Autodesk Fusion 360 part; units mm, degrees
(part 2 of 3)
  line L394 (91.6491, -63.7888) -> (96.0664, -64.6474)
  spline S217 degree 3 poles (106.4792, -50.6897) (105.7323, -50.6279) (105.0622, -51.1477) (104.9365, -51.8866) knots 0 0 0 0 1 1 1 1
  spline S218 degree 3 poles (7.9042, -66.3389) (7.576, -66.0107) (7.3916, -65.5656) (7.3916, -65.1015) knots 0 0 0 0 1 1 1 1
  spline S219 degree 3 poles (32.1681, -40.899) (31.7818, -41.2853) (31.2578, -41.5024) (30.7115, -41.5024) knots 0 0 0 0 1 1 1 1
  line L395 (26.4924, -39.9217) -> (26.4924, -39.9217)
  line L396 (96.8435, -63.2704) -> (97.4297, -62.875)
  line L397 (111.9353, -56.4836) -> (110.6261, -56.4379)
  spline S220 degree 3 poles (28.6515, -39.4424) (28.6515, -38.896) (28.8685, -38.372) (29.2548, -37.9857) knots 0 0 0 0 1 1 1 1
  line L398 (100.2141, -70.0378) -> (98.6435, -69.7326)
  spline S221 degree 3 poles (26.1234, -39.0308) (26.3597, -39.2671) (26.4924, -39.5875) (26.4924, -39.9217) knots 0 0 0 0 1 1 1 1
  spline S222 degree 3 poles (29.2548, -40.899) (28.8685, -40.5127) (28.6515, -39.9887) (28.6515, -39.4424) knots 0 0 0 0 1 1 1 1
  spline S223 degree 3 poles (36.1906, -40.223) (35.8564, -40.223) (35.5359, -40.0903) (35.2996, -39.854) knots 0 0 0 0 1 1 1 1
  line L399 (97.4297, -62.875) -> (102.3378, -63.829)
  line L400 (96.6527, -64.252) -> (96.8435, -63.2704)
  line L401 (103.1261, -76.3087) -> (101.8401, -76.0587)
  spline S224 degree 3 poles (103.4983, -45.9378) (103.5956, -45.8471) (103.6523, -45.721) (103.6556, -45.588) knots 0 0 0 0 1 1 1 1
  line L402 (31.7998, -44.3662) -> (30.4948, -44.4804)
  spline S225 degree 3 poles (37.0815, -38.072) (37.3178, -38.3083) (37.4506, -38.6288) (37.4506, -38.963) knots 0 0 0 0 1 1 1 1
  spline S226 degree 3 poles (7.3916, -65.1015) (7.3916, -64.6373) (7.576, -64.1922) (7.9042, -63.864) knots 0 0 0 0 1 1 1 1
  spline S227 degree 3 poles (112.8027, -57.4145) (112.8201, -56.918) (112.4318, -56.5013) (111.9353, -56.4836) knots 0 0 0 0 1 1 1 1
  spline S228 degree 3 poles (10.3791, -63.864) (10.7073, -64.1922) (10.8916, -64.6373) (10.8916, -65.1015) knots 0 0 0 0 1 1 1 1
  line L403 (102.749, -64.4387) -> (102.6575, -64.9098)
  spline S229 degree 3 poles (111.584, -35.6994) (111.8203, -35.4631) (112.1408, -35.3303) (112.4749, -35.3303) knots 0 0 0 0 1 1 1 1
  line L404 (38.9322, -55.8983) -> (38.9322, -55.8983)
  spline S230 degree 3 poles (29.2548, -37.9857) (29.6412, -37.5994) (30.1651, -37.3824) (30.7115, -37.3824) knots 0 0 0 0 1 1 1 1
  line L405 (32.7715, -39.4424) -> (32.7715, -39.4424)
  spline S231 degree 3 poles (37.6722, -57.1583) (37.338, -57.1583) (37.0175, -57.0256) (36.7812, -56.7893) knots 0 0 0 0 1 1 1 1
  spline S232 degree 3 poles (107.3956, -43.2171) (107.8921, -43.2341) (108.3085, -42.8455) (108.3258, -42.349) knots 0 0 0 0 1 1 1 1
  spline S233 degree 3 poles (85.5554, -23.6785) (85.6511, -23.5861) (85.7056, -23.4591) (85.7065, -23.3261) knots 0 0 0 0 1 1 1 1
  spline S234 degree 3 poles (111.2149, -36.5903) (111.2149, -36.2562) (111.3477, -35.9357) (111.584, -35.6994) knots 0 0 0 0 1 1 1 1
  spline S235 degree 3 poles (32.1681, -37.9857) (32.5545, -38.372) (32.7715, -38.896) (32.7715, -39.4424) knots 0 0 0 0 1 1 1 1
  spline S236 degree 3 poles (36.7812, -55.0074) (37.0175, -54.7711) (37.338, -54.6383) (37.6722, -54.6383) knots 0 0 0 0 1 1 1 1
  spline S237 degree 3 poles (85.1979, -23.8173) (85.3309, -23.8209) (85.4597, -23.7709) (85.5554, -23.6785) knots 0 0 0 0 1 1 1 1
  spline S238 degree 3 poles (33.6498, -54.921) (34.0361, -55.3074) (34.2531, -55.8313) (34.2531, -56.3777) knots 0 0 0 0 1 1 1 1
  spline S239 degree 3 poles (30.7115, -41.5024) (30.1651, -41.5024) (29.6412, -41.2853) (29.2548, -40.899) knots 0 0 0 0 1 1 1 1
  line L406 (85.724, -22.3262) -> (86.2326, -21.835)
  line L407 (107.4584, -41.4182) -> (106.1492, -41.3725)
  line L408 (87.0806, -30.5511) -> (87.0972, -29.6013)
  spline S240 degree 3 poles (113.7349, -36.5903) (113.7349, -36.9245) (113.6022, -37.245) (113.3659, -37.4813) knots 0 0 0 0 1 1 1 1
  line L409 (94.2137, -27.5752) -> (91.1841, -27.5223)
  line L410 (85.7065, -23.3261) -> (85.724, -22.3262)
  spline S241 degree 3 poles (30.7365, -54.921) (31.1228, -54.5347) (31.6468, -54.3177) (32.1931, -54.3177) knots 0 0 0 0 1 1 1 1
  spline S242 degree 3 poles (105.219, -42.2406) (105.2016, -42.7371) (105.5899, -43.1537) (106.0864, -43.1714) knots 0 0 0 0 1 1 1 1
  line L411 (34.2531, -56.3777) -> (34.2531, -56.3777)
  spline S243 degree 3 poles (38.5632, -56.7893) (38.3269, -57.0256) (38.0064, -57.1583) (37.6722, -57.1583) knots 0 0 0 0 1 1 1 1
  line L412 (86.2326, -21.835) -> (91.2319, -21.9223)
  spline S244 degree 3 poles (38.9322, -55.8983) (38.9322, -56.2325) (38.7995, -56.553) (38.5632, -56.7893) knots 0 0 0 0 1 1 1 1
  line L413 (90.2186, -28.4056) -> (88.6188, -28.3777)
  spline S245 degree 3 poles (30.7115, -37.3824) (31.2578, -37.3824) (31.7818, -37.5994) (32.1681, -37.9857) knots 0 0 0 0 1 1 1 1
  line L414 (91.1841, -27.5223) -> (90.2186, -28.4056)
  line L415 (87.0806, -30.5511) -> (80.5816, -30.4377)
  spline S246 degree 3 poles (106.1492, -41.3725) (105.6527, -41.3555) (105.2363, -41.744) (105.219, -42.2406) knots 0 0 0 0 1 1 1 1
  line L416 (80.5982, -29.4878) -> (78.0236, -29.4429)
  line L417 (78.0236, -29.4429) -> (78.1039, -24.8436)
  spline S247 degree 3 poles (37.6722, -54.6383) (38.0064, -54.6383) (38.3269, -54.7711) (38.5632, -55.0074) knots 0 0 0 0 1 1 1 1
  spline S248 degree 3 poles (113.3659, -37.4813) (113.1296, -37.7176) (112.8091, -37.8503) (112.4749, -37.8503) knots 0 0 0 0 1 1 1 1
  line L418 (80.6986, -23.7387) -> (85.1979, -23.8173)
  spline S249 degree 3 poles (89.4046, -20.8902) (89.9013, -20.8984) (90.3106, -20.5027) (90.3193, -20.0061) knots 0 0 0 0 1 1 1 1
  spline S250 degree 3 poles (88.6188, -28.3777) (87.8709, -28.3289) (87.21, -28.8604) (87.0972, -29.6013) knots 0 0 0 0 1 1 1 1
  line L419 (89.4046, -20.8902) -> (88.0948, -20.8674)
  spline S251 degree 3 poles (90.3193, -20.0061) (90.328, -19.5094) (89.9326, -19.0997) (89.436, -19.0905) knots 0 0 0 0 1 1 1 1
  spline S252 degree 3 poles (87.2115, -19.9518) (87.2029, -20.4485) (87.5982, -20.8582) (88.0948, -20.8674) knots 0 0 0 0 1 1 1 1
  spline S253 degree 3 poles (111.584, -37.4813) (111.3477, -37.245) (111.2149, -36.9245) (111.2149, -36.5903) knots 0 0 0 0 1 1 1 1
  spline S254 degree 3 poles (88.1262, -19.0676) (87.6296, -19.0595) (87.2202, -19.4552) (87.2115, -19.9518) knots 0 0 0 0 1 1 1 1
  spline S255 degree 3 poles (112.4749, -37.8503) (112.1408, -37.8503) (111.8203, -37.7176) (111.584, -37.4813) knots 0 0 0 0 1 1 1 1
  spline S256 degree 3 poles (36.4122, -55.8983) (36.4122, -55.5641) (36.545, -55.2437) (36.7812, -55.0074) knots 0 0 0 0 1 1 1 1
  line L420 (80.5816, -30.4377) -> (80.5982, -29.4878)
  spline S257 degree 3 poles (38.5632, -55.0074) (38.7995, -55.2437) (38.9322, -55.5641) (38.9322, -55.8983) knots 0 0 0 0 1 1 1 1
  line L421 (107.3956, -43.2171) -> (106.0864, -43.1714)
  line L422 (80.6785, -24.8885) -> (80.6986, -23.7387)
  line L423 (78.1039, -24.8436) -> (80.6785, -24.8885)
  line L424 (91.7343, -22.9312) -> (94.294, -22.9759)
  spline S258 degree 3 poles (108.3258, -42.349) (108.3431, -41.8525) (107.9549, -41.4359) (107.4584, -41.4182) knots 0 0 0 0 1 1 1 1
  spline S259 degree 3 poles (90.9284, -14.0798) (90.9284, -14.6262) (90.7113, -15.1501) (90.325, -15.5365) knots 0 0 0 0 1 1 1 1
  spline S260 degree 3 poles (90.325, -15.5365) (89.9387, -15.9228) (89.4147, -16.1398) (88.8684, -16.1398) knots 0 0 0 0 1 1 1 1
  line L425 (91.7427, -22.4513) -> (91.7343, -22.9312)
  spline S261 degree 3 poles (36.7812, -56.7893) (36.545, -56.553) (36.4122, -56.2325) (36.4122, -55.8983) knots 0 0 0 0 1 1 1 1
  line L426 (94.2137, -27.5752) -> (94.294, -22.9759)
  spline S262 degree 3 poles (88.8684, -16.1398) (88.322, -16.1398) (87.7981, -15.9228) (87.4117, -15.5365) knots 0 0 0 0 1 1 1 1
  spline S263 degree 3 poles (87.4117, -15.5365) (87.0254, -15.1501) (86.8084, -14.6262) (86.8084, -14.0798) knots 0 0 0 0 1 1 1 1
  spline S264 degree 3 poles (88.8684, -12.0198) (89.4147, -12.0198) (89.9387, -12.2369) (90.325, -12.6232) knots 0 0 0 0 1 1 1 1
  spline S265 degree 3 poles (86.8084, -14.0798) (86.8084, -12.9421) (87.7307, -12.0198) (88.8684, -12.0198) knots 0 0 0 0 1 1 1 1
  spline S266 degree 3 poles (32.1931, -54.3177) (32.7395, -54.3177) (33.2634, -54.5347) (33.6498, -54.921) knots 0 0 0 0 1 1 1 1
  line L427 (89.436, -19.0905) -> (88.1262, -19.0676)
  line L428 (91.2319, -21.9223) -> (91.7427, -22.4513)
  spline S267 degree 3 poles (82.1092, -13.9838) (82.1092, -13.6497) (82.242, -13.3292) (82.4783, -13.0929) knots 0 0 0 0 1 1 1 1
  spline S268 degree 3 poles (94.0709, -32.4332) (93.7367, -32.4332) (93.4162, -32.3005) (93.1799, -32.0642) knots 0 0 0 0 1 1 1 1
  line L429 (95.3309, -31.1732) -> (95.3309, -31.1732)
  spline S269 degree 3 poles (94.9618, -30.2823) (95.1981, -30.5186) (95.3309, -30.8391) (95.3309, -31.1732) knots 0 0 0 0 1 1 1 1
  spline S270 degree 3 poles (11.2142, -14.5989) (10.886, -14.2707) (10.7016, -13.8256) (10.7016, -13.3615) knots 0 0 0 0 1 1 1 1
  spline S271 degree 3 poles (11.2142, -12.124) (11.5424, -11.7958) (11.9875, -11.6115) (12.4516, -11.6115) knots 0 0 0 0 1 1 1 1
  spline S272 degree 3 poles (10.3791, -66.3389) (10.0509, -66.6671) (9.6058, -66.8515) (9.1416, -66.8515) knots 0 0 0 0 1 1 1 1
  spline S273 degree 3 poles (84.6292, -13.9838) (84.6292, -14.318) (84.4965, -14.6385) (84.2602, -14.8748) knots 0 0 0 0 1 1 1 1
  spline S274 degree 3 poles (90.6317, -31.0772) (90.6317, -31.6236) (90.4147, -32.1476) (90.0283, -32.5339) knots 0 0 0 0 1 1 1 1
  spline S275 degree 3 poles (93.4766, -13.2849) (93.7129, -13.0486) (94.0334, -12.9158) (94.3675, -12.9158) knots 0 0 0 0 1 1 1 1
  spline S276 degree 3 poles (88.5717, -29.0172) (89.118, -29.0172) (89.642, -29.2343) (90.0283, -29.6206) knots 0 0 0 0 1 1 1 1
  line L430 (89.1393, -36.0879) -> (87.8295, -36.0651)
  spline S277 degree 3 poles (88.5717, -33.1372) (88.0254, -33.1372) (87.5014, -32.9202) (87.1151, -32.5339) knots 0 0 0 0 1 1 1 1
  spline S278 degree 3 poles (81.8125, -30.9813) (81.8125, -30.6471) (81.9453, -30.3266) (82.1816, -30.0903) knots 0 0 0 0 1 1 1 1
  spline S279 degree 3 poles (87.1151, -29.6206) (87.5014, -29.2343) (88.0254, -29.0172) (88.5717, -29.0172) knots 0 0 0 0 1 1 1 1
  line L431 (90.9284, -14.0798) -> (90.9284, -14.0798)
  line L432 (90.6317, -31.0772) -> (90.6317, -31.0772)
  spline S280 degree 3 poles (95.2585, -13.2849) (95.4948, -13.5212) (95.6275, -13.8416) (95.6275, -14.1758) knots 0 0 0 0 1 1 1 1
  line L433 (84.6292, -13.9838) -> (84.6292, -13.9838)
  spline S281 degree 3 poles (94.0709, -29.9132) (94.405, -29.9132) (94.7255, -30.046) (94.9618, -30.2823) knots 0 0 0 0 1 1 1 1
  spline S282 degree 3 poles (10.7016, -13.3615) (10.7016, -12.8973) (10.886, -12.4522) (11.2142, -12.124) knots 0 0 0 0 1 1 1 1
  spline S283 degree 3 poles (14.8422, -46.7533) (14.7989, -46.2586) (14.363, -45.8924) (13.8683, -45.935) knots 0 0 0 0 1 1 1 1
  spline S284 degree 3 poles (83.3692, -15.2438) (83.0351, -15.2438) (82.7146, -15.1111) (82.4783, -14.8748) knots 0 0 0 0 1 1 1 1
  spline S285 degree 3 poles (94.3675, -15.4358) (94.0334, -15.4358) (93.7129, -15.3031) (93.4766, -15.0668) knots 0 0 0 0 1 1 1 1
  spline S286 degree 3 poles (9.1416, -66.8515) (8.6775, -66.8515) (8.2324, -66.6671) (7.9042, -66.3389) knots 0 0 0 0 1 1 1 1
  spline S287 degree 3 poles (10.8916, -65.1015) (10.8916, -65.5656) (10.7073, -66.0107) (10.3791, -66.3389) knots 0 0 0 0 1 1 1 1
  spline S288 degree 3 poles (89.1079, -37.8876) (89.6046, -37.8958) (90.0139, -37.5001) (90.0226, -37.0035) knots 0 0 0 0 1 1 1 1
  spline S289 degree 3 poles (86.9148, -36.9492) (86.9062, -37.4459) (87.3015, -37.8556) (87.7981, -37.8648) knots 0 0 0 0 1 1 1 1
  spline S290 degree 3 poles (82.1816, -30.0903) (82.4179, -29.854) (82.7384, -29.7213) (83.0725, -29.7213) knots 0 0 0 0 1 1 1 1
  spline S291 degree 3 poles (94.9618, -32.0642) (94.7255, -32.3005) (94.405, -32.4332) (94.0709, -32.4332) knots 0 0 0 0 1 1 1 1
  spline S292 degree 3 poles (95.2585, -15.0668) (95.0222, -15.3031) (94.7017, -15.4358) (94.3675, -15.4358) knots 0 0 0 0 1 1 1 1
  spline S293 degree 3 poles (90.325, -12.6232) (90.7113, -13.0095) (90.9284, -13.5335) (90.9284, -14.0798) knots 0 0 0 0 1 1 1 1
  spline S294 degree 3 poles (82.1816, -31.8722) (81.9453, -31.6359) (81.8125, -31.3154) (81.8125, -30.9813) knots 0 0 0 0 1 1 1 1
  spline S295 degree 3 poles (93.1799, -30.2823) (93.4162, -30.046) (93.7367, -29.9132) (94.0709, -29.9132) knots 0 0 0 0 1 1 1 1
  spline S296 degree 3 poles (83.9635, -31.8722) (83.7272, -32.1085) (83.4067, -32.2413) (83.0725, -32.2413) knots 0 0 0 0 1 1 1 1
  spline S297 degree 3 poles (82.4783, -13.0929) (82.7146, -12.8566) (83.0351, -12.7238) (83.3692, -12.7238) knots 0 0 0 0 1 1 1 1
  spline S298 degree 3 poles (84.3325, -30.9813) (84.3325, -31.3154) (84.1998, -31.6359) (83.9635, -31.8722) knots 0 0 0 0 1 1 1 1
  spline S299 degree 3 poles (83.0725, -29.7213) (83.4067, -29.7213) (83.7272, -29.854) (83.9635, -30.0903) knots 0 0 0 0 1 1 1 1
  spline S300 degree 3 poles (87.1151, -32.5339) (86.7287, -32.1476) (86.5117, -31.6236) (86.5117, -31.0772) knots 0 0 0 0 1 1 1 1
  spline S301 degree 3 poles (95.6275, -14.1758) (95.6275, -14.51) (95.4948, -14.8305) (95.2585, -15.0668) knots 0 0 0 0 1 1 1 1
  spline S302 degree 3 poles (92.8109, -31.1732) (92.8109, -30.8391) (92.9436, -30.5186) (93.1799, -30.2823) knots 0 0 0 0 1 1 1 1
  spline S303 degree 3 poles (83.0725, -32.2413) (82.7384, -32.2413) (82.4179, -32.1085) (82.1816, -31.8722) knots 0 0 0 0 1 1 1 1
  line L434 (95.6275, -14.1758) -> (95.6275, -14.1758)
  spline S304 degree 3 poles (14.2016, -13.3615) (14.2016, -14.328) (13.4181, -15.1115) (12.4516, -15.1115) knots 0 0 0 0 1 1 1 1
  spline S305 degree 3 poles (12.4516, -15.1115) (11.9875, -15.1115) (11.5424, -14.9271) (11.2142, -14.5989) knots 0 0 0 0 1 1 1 1
  spline S306 degree 3 poles (12.4516, -11.6115) (13.4181, -11.6115) (14.2016, -12.395) (14.2016, -13.3615) knots 0 0 0 0 1 1 1 1
  spline S307 degree 3 poles (90.0283, -32.5339) (89.642, -32.9202) (89.118, -33.1372) (88.5717, -33.1372) knots 0 0 0 0 1 1 1 1
  line L435 (14.2016, -13.3615) -> (14.2016, -13.3615)
  spline S308 degree 3 poles (14.0251, -47.7282) (14.5198, -47.6843) (14.8854, -47.248) (14.8422, -46.7533) knots 0 0 0 0 1 1 1 1
  spline S309 degree 3 poles (82.4783, -14.8748) (82.242, -14.6385) (82.1092, -14.318) (82.1092, -13.9838) knots 0 0 0 0 1 1 1 1
  spline S310 degree 3 poles (84.2602, -13.0929) (84.4965, -13.3292) (84.6292, -13.6497) (84.6292, -13.9838) knots 0 0 0 0 1 1 1 1
  spline S311 degree 3 poles (90.0226, -37.0035) (90.0313, -36.5068) (89.636, -36.0971) (89.1393, -36.0879) knots 0 0 0 0 1 1 1 1
  spline S312 degree 3 poles (84.2602, -14.8748) (84.0239, -15.1111) (83.7034, -15.2438) (83.3692, -15.2438) knots 0 0 0 0 1 1 1 1
  spline S313 degree 3 poles (93.1075, -14.1758) (93.1075, -13.8416) (93.2403, -13.5212) (93.4766, -13.2849) knots 0 0 0 0 1 1 1 1
  line L436 (89.1079, -37.8876) -> (87.7981, -37.8648)
  spline S314 degree 3 poles (86.5117, -31.0772) (86.5117, -30.5309) (86.7287, -30.0069) (87.1151, -29.6206) knots 0 0 0 0 1 1 1 1
  spline S315 degree 3 poles (94.3675, -12.9158) (94.7017, -12.9158) (95.0222, -13.0486) (95.2585, -13.2849) knots 0 0 0 0 1 1 1 1
  line L437 (84.3325, -30.9813) -> (84.3325, -30.9813)
  spline S316 degree 3 poles (83.3692, -12.7238) (83.7034, -12.7238) (84.0239, -12.8566) (84.2602, -13.0929) knots 0 0 0 0 1 1 1 1
  spline S317 degree 3 poles (95.3309, -31.1732) (95.3309, -31.5074) (95.1981, -31.8279) (94.9618, -32.0642) knots 0 0 0 0 1 1 1 1
  spline S318 degree 3 poles (83.9635, -30.0903) (84.1998, -30.3266) (84.3325, -30.6471) (84.3325, -30.9813) knots 0 0 0 0 1 1 1 1
  spline S319 degree 3 poles (93.4766, -15.0668) (93.2403, -14.8305) (93.1075, -14.51) (93.1075, -14.1758) knots 0 0 0 0 1 1 1 1
  spline S320 degree 3 poles (90.0283, -29.6206) (90.4147, -30.0069) (90.6317, -30.5309) (90.6317, -31.0772) knots 0 0 0 0 1 1 1 1
  spline S321 degree 3 poles (93.1799, -32.0642) (92.9436, -31.8279) (92.8109, -31.5074) (92.8109, -31.1732) knots 0 0 0 0 1 1 1 1
  line L438 (13.8683, -45.935) -> (12.5633, -46.0492)
  spline S322 degree 3 poles (7.3009, -42.7505) (6.9667, -42.7505) (6.6463, -42.6178) (6.41, -42.3815) knots 0 0 0 0 1 1 1 1
  spline S323 degree 3 poles (14.84, -41.0112) (14.84, -41.5575) (14.6229, -42.0815) (14.2366, -42.4678) knots 0 0 0 0 1 1 1 1
  spline S324 degree 3 poles (10.72, -41.0112) (10.72, -40.4648) (10.937, -39.9408) (11.3233, -39.5545) knots 0 0 0 0 1 1 1 1
  spline S325 degree 3 poles (12.78, -38.9512) (13.3263, -38.9512) (13.8503, -39.1682) (14.2366, -39.5545) knots 0 0 0 0 1 1 1 1
  line L439 (19.5191, -40.5318) -> (19.5191, -40.5318)
  spline S326 degree 3 poles (11.3233, -42.4678) (10.937, -42.0815) (10.72, -41.5575) (10.72, -41.0112) knots 0 0 0 0 1 1 1 1
  spline S327 degree 3 poles (111.3791, -71.7789) (111.0509, -72.1071) (110.6058, -72.2915) (110.1416, -72.2915) knots 0 0 0 0 1 1 1 1
  spline S328 degree 3 poles (110.1416, -68.7915) (110.6058, -68.7915) (111.0509, -68.9758) (111.3791, -69.304) knots 0 0 0 0 1 1 1 1
  spline S329 degree 3 poles (108.9042, -69.304) (109.2324, -68.9758) (109.6775, -68.7915) (110.1416, -68.7915) knots 0 0 0 0 1 1 1 1
  spline S330 degree 3 poles (12.78, -43.0712) (12.2336, -43.0712) (11.7097, -42.8541) (11.3233, -42.4678) knots 0 0 0 0 1 1 1 1
  spline S331 degree 3 poles (8.1919, -40.5996) (8.4282, -40.8359) (8.5609, -41.1563) (8.5609, -41.4905) knots 0 0 0 0 1 1 1 1
  spline S332 degree 3 poles (18.2591, -39.2718) (18.5932, -39.2718) (18.9137, -39.4046) (19.15, -39.6409) knots 0 0 0 0 1 1 1 1
  spline S333 degree 3 poles (11.7462, -47.0241) (11.7895, -47.5189) (12.2254, -47.885) (12.7201, -47.8424) knots 0 0 0 0 1 1 1 1
  spline S334 degree 3 poles (111.8916, -70.5415) (111.8916, -71.0056) (111.7073, -71.4507) (111.3791, -71.7789) knots 0 0 0 0 1 1 1 1
  spline S335 degree 3 poles (108.3916, -70.5415) (108.3916, -70.0773) (108.576, -69.6322) (108.9042, -69.304) knots 0 0 0 0 1 1 1 1
  spline S336 degree 3 poles (111.3791, -69.304) (111.7073, -69.6322) (111.8916, -70.0773) (111.8916, -70.5415) knots 0 0 0 0 1 1 1 1
  line L440 (111.8916, -70.5415) -> (111.8916, -70.5415)
  spline S337 degree 3 poles (33.4383, -63.0947) (33.933, -63.0508) (34.2986, -62.6145) (34.2553, -62.1198) knots 0 0 0 0 1 1 1 1
  spline S338 degree 3 poles (11.3233, -39.5545) (11.7097, -39.1682) (12.2336, -38.9512) (12.78, -38.9512) knots 0 0 0 0 1 1 1 1
  spline S339 degree 3 poles (110.1416, -72.2915) (109.1751, -72.2915) (108.3916, -71.508) (108.3916, -70.5415) knots 0 0 0 0 1 1 1 1
  spline S340 degree 3 poles (31.9764, -61.4157) (31.4817, -61.4596) (31.1161, -61.8959) (31.1594, -62.3906) knots 0 0 0 0 1 1 1 1
  spline S341 degree 3 poles (14.2366, -39.5545) (14.6229, -39.9408) (14.84, -40.4648) (14.84, -41.0112) knots 0 0 0 0 1 1 1 1
  spline S342 degree 3 poles (19.5191, -40.5318) (19.5191, -40.866) (19.3863, -41.1865) (19.15, -41.4228) knots 0 0 0 0 1 1 1 1
  line L441 (14.0251, -47.7282) -> (12.7201, -47.8424)
  spline S343 degree 3 poles (8.1919, -42.3815) (7.9556, -42.6178) (7.6351, -42.7505) (7.3009, -42.7505) knots 0 0 0 0 1 1 1 1
  spline S344 degree 3 poles (6.41, -42.3815) (6.1737, -42.1452) (6.0409, -41.8247) (6.0409, -41.4905) knots 0 0 0 0 1 1 1 1
  spline S345 degree 3 poles (14.2366, -42.4678) (13.8503, -42.8541) (13.3263, -43.0712) (12.78, -43.0712) knots 0 0 0 0 1 1 1 1
  spline S346 degree 3 poles (6.41, -40.5996) (6.6463, -40.3633) (6.9667, -40.2305) (7.3009, -40.2305) knots 0 0 0 0 1 1 1 1
  line L442 (8.5609, -41.4905) -> (8.5609, -41.4905)
  line L443 (14.84, -41.0112) -> (14.84, -41.0112)
  spline S347 degree 3 poles (18.2591, -41.7918) (17.9249, -41.7918) (17.6044, -41.6591) (17.3681, -41.4228) knots 0 0 0 0 1 1 1 1
  spline S348 degree 3 poles (17.3681, -41.4228) (17.1318, -41.1865) (16.9991, -40.866) (16.9991, -40.5318) knots 0 0 0 0 1 1 1 1
  spline S349 degree 3 poles (8.5609, -41.4905) (8.5609, -41.8247) (8.4282, -42.1452) (8.1919, -42.3815) knots 0 0 0 0 1 1 1 1
  spline S350 degree 3 poles (12.5633, -46.0492) (12.0686, -46.0931) (11.703, -46.5294) (11.7462, -47.0241) knots 0 0 0 0 1 1 1 1
  spline S351 degree 3 poles (19.15, -41.4228) (18.9137, -41.6591) (18.5932, -41.7918) (18.2591, -41.7918) knots 0 0 0 0 1 1 1 1
  spline S352 degree 3 poles (6.0409, -41.4905) (6.0409, -41.1563) (6.1737, -40.8359) (6.41, -40.5996) knots 0 0 0 0 1 1 1 1
  spline S353 degree 3 poles (16.9991, -40.5318) (16.9991, -40.1976) (17.1318, -39.8771) (17.3681, -39.6409) knots 0 0 0 0 1 1 1 1
  spline S354 degree 3 poles (19.15, -39.6409) (19.3863, -39.8771) (19.5191, -40.1976) (19.5191, -40.5318) knots 0 0 0 0 1 1 1 1
  spline S355 degree 3 poles (17.3681, -39.6409) (17.6044, -39.4046) (17.9249, -39.2718) (18.2591, -39.2718) knots 0 0 0 0 1 1 1 1
  spline S356 degree 3 poles (7.3009, -40.2305) (7.6351, -40.2305) (7.9556, -40.3633) (8.1919, -40.5996) knots 0 0 0 0 1 1 1 1
  spline S357 degree 3 poles (122.216, -74.966) (122.216, -75.5123) (121.999, -76.0363) (121.6127, -76.4226) knots 0 0 0 0 1 1 1 1
  line L444 (124.9371, -76.5691) -> (124.3629, -77.7465)
  spline S358 degree 3 poles (34.2531, -56.3777) (34.2531, -56.924) (34.0361, -57.448) (33.6498, -57.8343) knots 0 0 0 0 1 1 1 1
  spline S359 degree 3 poles (70.075, -26.0147) (70.6213, -26.0147) (71.1453, -26.2317) (71.5316, -26.618) knots 0 0 0 0 1 1 1 1
  spline S360 degree 3 poles (76.835, -28.0747) (76.835, -28.4088) (76.7023, -28.7293) (76.466, -28.9656) knots 0 0 0 0 1 1 1 1
  spline S361 degree 3 poles (76.466, -27.1837) (76.7023, -27.42) (76.835, -27.7405) (76.835, -28.0747) knots 0 0 0 0 1 1 1 1
  spline S362 degree 3 poles (33.6498, -57.8343) (33.2634, -58.2206) (32.7395, -58.4377) (32.1931, -58.4377) knots 0 0 0 0 1 1 1 1
  spline S363 degree 3 poles (71.5316, -26.618) (71.918, -27.0043) (72.135, -27.5283) (72.135, -28.0747) knots 0 0 0 0 1 1 1 1
  spline S364 degree 3 poles (74.684, -27.1837) (74.9203, -26.9474) (75.2408, -26.8147) (75.575, -26.8147) knots 0 0 0 0 1 1 1 1
  spline S365 degree 3 poles (75.575, -26.8147) (75.9092, -26.8147) (76.2297, -26.9474) (76.466, -27.1837) knots 0 0 0 0 1 1 1 1
  spline S366 degree 3 poles (126.1401, -76.1557) (125.6937, -75.938) (125.1554, -76.123) (124.9371, -76.5691) knots 0 0 0 0 1 1 1 1
  spline S367 degree 3 poles (122.5671, -68.7626) (122.9013, -68.7626) (123.2217, -68.8954) (123.458, -69.1317) knots 0 0 0 0 1 1 1 1
  spline S368 degree 3 poles (118.636, -79.0184) (118.8723, -79.2547) (119.005, -79.5752) (119.005, -79.9093) knots 0 0 0 0 1 1 1 1
  line L445 (119.005, -79.9093) -> (119.005, -79.9093)
  spline S369 degree 3 poles (121.6761, -69.1317) (121.9124, -68.8954) (122.2329, -68.7626) (122.5671, -68.7626) knots 0 0 0 0 1 1 1 1
  line L446 (72.135, -28.0747) -> (72.135, -28.0747)
  line L447 (76.835, -28.0747) -> (76.835, -28.0747)
  spline S370 degree 3 poles (118.6994, -76.4226) (118.3131, -76.0363) (118.096, -75.5123) (118.096, -74.966) knots 0 0 0 0 1 1 1 1
  spline S371 degree 3 poles (121.3071, -70.0226) (121.3071, -69.6884) (121.4398, -69.3679) (121.6761, -69.1317) knots 0 0 0 0 1 1 1 1
  spline S372 degree 3 poles (121.6761, -70.9136) (121.4398, -70.6773) (121.3071, -70.3568) (121.3071, -70.0226) knots 0 0 0 0 1 1 1 1
  spline S373 degree 3 poles (27.605, -55.9661) (27.8413, -56.2024) (27.9741, -56.5229) (27.9741, -56.857) knots 0 0 0 0 1 1 1 1
  spline S374 degree 3 poles (87.8295, -36.0651) (87.3329, -36.0569) (86.9235, -36.4526) (86.9148, -36.9492) knots 0 0 0 0 1 1 1 1
  spline S375 degree 3 poles (121.6127, -76.4226) (121.2264, -76.8089) (120.7024, -77.026) (120.156, -77.026) knots 0 0 0 0 1 1 1 1
  spline S376 degree 3 poles (126.555, -77.3582) (126.7721, -76.9116) (126.5865, -76.3734) (126.1401, -76.1557) knots 0 0 0 0 1 1 1 1
  spline S377 degree 3 poles (123.458, -69.1317) (123.6943, -69.3679) (123.8271, -69.6884) (123.8271, -70.0226) knots 0 0 0 0 1 1 1 1
  spline S378 degree 3 poles (25.8231, -57.748) (25.5868, -57.5117) (25.4541, -57.1912) (25.4541, -56.857) knots 0 0 0 0 1 1 1 1
  spline S379 degree 3 poles (26.7141, -55.597) (27.0482, -55.597) (27.3687, -55.7298) (27.605, -55.9661) knots 0 0 0 0 1 1 1 1
  spline S380 degree 3 poles (30.1331, -56.3777) (30.1331, -55.8313) (30.3502, -55.3074) (30.7365, -54.921) knots 0 0 0 0 1 1 1 1
  spline S381 degree 3 poles (74.684, -28.9656) (74.4477, -28.7293) (74.315, -28.4088) (74.315, -28.0747) knots 0 0 0 0 1 1 1 1
  line L448 (27.9741, -56.857) -> (27.9741, -56.857)
  line L449 (122.216, -74.966) -> (122.216, -74.966)
  spline S382 degree 3 poles (120.156, -72.906) (121.2937, -72.906) (122.216, -73.8283) (122.216, -74.966) knots 0 0 0 0 1 1 1 1
  line L450 (33.2814, -61.3016) -> (31.9764, -61.4157)
  spline S383 degree 3 poles (25.4541, -56.857) (25.4541, -56.5229) (25.5868, -56.2024) (25.8231, -55.9661) knots 0 0 0 0 1 1 1 1
  spline S384 degree 3 poles (118.096, -74.966) (118.096, -74.4196) (118.3131, -73.8957) (118.6994, -73.5093) knots 0 0 0 0 1 1 1 1
  spline S385 degree 3 poles (117.745, -81.1693) (117.4108, -81.1693) (117.0903, -81.0366) (116.854, -80.8003) knots 0 0 0 0 1 1 1 1
  spline S386 degree 3 poles (27.605, -57.748) (27.3687, -57.9843) (27.0482, -58.117) (26.7141, -58.117) knots 0 0 0 0 1 1 1 1
  spline S387 degree 3 poles (27.9741, -56.857) (27.9741, -57.1912) (27.8413, -57.5117) (27.605, -57.748) knots 0 0 0 0 1 1 1 1
  spline S388 degree 3 poles (119.005, -79.9093) (119.005, -80.2435) (118.8723, -80.564) (118.636, -80.8003) knots 0 0 0 0 1 1 1 1
  spline S389 degree 3 poles (116.485, -79.9093) (116.485, -79.5752) (116.6178, -79.2547) (116.854, -79.0184) knots 0 0 0 0 1 1 1 1
  spline S390 degree 3 poles (117.745, -78.6493) (118.0792, -78.6493) (118.3997, -78.7821) (118.636, -79.0184) knots 0 0 0 0 1 1 1 1
  spline S391 degree 3 poles (123.458, -70.9136) (123.2217, -71.1499) (122.9013, -71.2826) (122.5671, -71.2826) knots 0 0 0 0 1 1 1 1
  spline S392 degree 3 poles (122.5671, -71.2826) (122.2329, -71.2826) (121.9124, -71.1499) (121.6761, -70.9136) knots 0 0 0 0 1 1 1 1
  spline S393 degree 3 poles (32.1931, -58.4377) (31.6468, -58.4377) (31.1228, -58.2206) (30.7365, -57.8343) knots 0 0 0 0 1 1 1 1
  spline S394 degree 3 poles (76.466, -28.9656) (76.2297, -29.2019) (75.9092, -29.3347) (75.575, -29.3347) knots 0 0 0 0 1 1 1 1
  spline S395 degree 3 poles (123.8271, -70.0226) (123.8271, -70.3568) (123.6943, -70.6773) (123.458, -70.9136) knots 0 0 0 0 1 1 1 1
  spline S396 degree 3 poles (25.8231, -55.9661) (26.0594, -55.7298) (26.3799, -55.597) (26.7141, -55.597) knots 0 0 0 0 1 1 1 1
  spline S397 degree 3 poles (120.156, -77.026) (119.6097, -77.026) (119.0857, -76.8089) (118.6994, -76.4226) knots 0 0 0 0 1 1 1 1
  line L451 (33.4383, -63.0947) -> (32.1333, -63.2089)
  spline S398 degree 3 poles (75.575, -29.3347) (75.2408, -29.3347) (74.9203, -29.2019) (74.684, -28.9656) knots 0 0 0 0 1 1 1 1
  spline S399 degree 3 poles (34.2553, -62.1198) (34.212, -61.6251) (33.7762, -61.2589) (33.2814, -61.3016) knots 0 0 0 0 1 1 1 1
  spline S400 degree 3 poles (26.7141, -58.117) (26.3799, -58.117) (26.0594, -57.9843) (25.8231, -57.748) knots 0 0 0 0 1 1 1 1
  spline S401 degree 3 poles (124.3629, -77.7465) (124.1468, -78.193) (124.3327, -78.7301) (124.7785, -78.9475) knots 0 0 0 0 1 1 1 1
  line L452 (123.8271, -70.0226) -> (123.8271, -70.0226)
  spline S402 degree 3 poles (124.7785, -78.9475) (125.2242, -79.1649) (125.7619, -78.9807) (125.9807, -78.5356) knots 0 0 0 0 1 1 1 1
  line L453 (126.555, -77.3582) -> (125.9807, -78.5356)
  spline S403 degree 3 poles (74.315, -28.0747) (74.315, -27.7405) (74.4477, -27.42) (74.684, -27.1837) knots 0 0 0 0 1 1 1 1
  spline S404 degree 3 poles (118.6994, -73.5093) (119.0857, -73.123) (119.6097, -72.906) (120.156, -72.906) knots 0 0 0 0 1 1 1 1
  spline S405 degree 3 poles (118.636, -80.8003) (118.3997, -81.0366) (118.0792, -81.1693) (117.745, -81.1693) knots 0 0 0 0 1 1 1 1
  spline S406 degree 3 poles (116.854, -80.8003) (116.6178, -80.564) (116.485, -80.2435) (116.485, -79.9093) knots 0 0 0 0 1 1 1 1
  spline S407 degree 3 poles (116.854, -79.0184) (117.0903, -78.7821) (117.4108, -78.6493) (117.745, -78.6493) knots 0 0 0 0 1 1 1 1
  line L454 (72.2816, -72.7915) -> (72.2816, -72.7915)
  spline S408 degree 3 poles (31.1594, -62.3906) (31.2027, -62.8854) (31.6385, -63.2515) (32.1333, -63.2089) knots 0 0 0 0 1 1 1 1
  spline S409 degree 3 poles (30.7365, -57.8343) (30.3502, -57.448) (30.1331, -56.924) (30.1331, -56.3777) knots 0 0 0 0 1 1 1 1
  spline S410 degree 3 poles (49.1114, -53.0828) (49.1374, -53.5788) (49.5602, -53.9599) (50.0563, -53.9345) knots 0 0 0 0 1 1 1 1
  spline S411 degree 3 poles (49.962, -52.137) (49.4661, -52.1635) (49.0854, -52.5868) (49.1114, -53.0828) knots 0 0 0 0 1 1 1 1
  spline S412 degree 3 poles (52.2151, -52.9201) (52.1891, -52.4241) (51.7663, -52.043) (51.2703, -52.0684) knots 0 0 0 0 1 1 1 1
  spline S413 degree 3 poles (71.5316, -29.5313) (71.1453, -29.9176) (70.6213, -30.1347) (70.075, -30.1347) knots 0 0 0 0 1 1 1 1
  spline S414 degree 3 poles (46.122, -47.3974) (46.122, -47.7316) (45.9893, -48.052) (45.753, -48.2883) knots 0 0 0 0 1 1 1 1
  spline S415 degree 3 poles (55.8469, -45.5617) (56.1811, -45.5617) (56.5016, -45.6944) (56.7379, -45.9307) knots 0 0 0 0 1 1 1 1
  spline S416 degree 3 poles (70.075, -30.1347) (69.5287, -30.1347) (69.0047, -29.9176) (68.6184, -29.5313) knots 0 0 0 0 1 1 1 1
  spline S417 degree 3 poles (69.42, -33.0747) (69.0985, -33.0747) (68.8013, -33.2462) (68.6406, -33.5247) knots 0 0 0 0 1 1 1 1
  spline S418 degree 3 poles (51.8111, -45.6529) (52.1974, -46.0392) (52.4145, -46.5632) (52.4145, -47.1095) knots 0 0 0 0 1 1 1 1
  spline S419 degree 3 poles (132.6091, -60.524) (132.9373, -60.8522) (133.1216, -61.2973) (133.1216, -61.7615) knots 0 0 0 0 1 1 1 1
  spline S420 degree 3 poles (43.9711, -46.5064) (44.2073, -46.2701) (44.5278, -46.1374) (44.862, -46.1374) knots 0 0 0 0 1 1 1 1
  line L455 (133.1216, -61.7615) -> (133.1216, -61.7615)
  spline S421 degree 3 poles (44.862, -46.1374) (45.1962, -46.1374) (45.5167, -46.2701) (45.753, -46.5064) knots 0 0 0 0 1 1 1 1
  spline S422 degree 3 poles (131.3716, -60.0115) (131.8358, -60.0115) (132.2809, -60.1958) (132.6091, -60.524) knots 0 0 0 0 1 1 1 1
  spline S423 degree 3 poles (48.8978, -48.5662) (48.5115, -48.1799) (48.2945, -47.6559) (48.2945, -47.1095) knots 0 0 0 0 1 1 1 1
  spline S424 degree 3 poles (70.5316, -71.0415) (70.9958, -71.0415) (71.4409, -71.2258) (71.7691, -71.554) knots 0 0 0 0 1 1 1 1
  line L456 (51.3645, -53.8659) -> (50.0563, -53.9345)
  line L457 (46.122, -47.3974) -> (46.122, -47.3974)
  spline S425 degree 3 poles (55.8469, -48.0817) (55.5128, -48.0817) (55.1923, -47.9489) (54.956, -47.7126) knots 0 0 0 0 1 1 1 1
  spline S426 degree 3 poles (56.7379, -45.9307) (56.9742, -46.167) (57.1069, -46.4875) (57.1069, -46.8217) knots 0 0 0 0 1 1 1 1
  spline S427 degree 3 poles (48.2945, -47.1095) (48.2945, -46.5632) (48.5115, -46.0392) (48.8978, -45.6529) knots 0 0 0 0 1 1 1 1
  spline S428 degree 3 poles (71.7691, -71.554) (72.0973, -71.8822) (72.2816, -72.3273) (72.2816, -72.7915) knots 0 0 0 0 1 1 1 1
  spline S429 degree 3 poles (50.3545, -45.0495) (50.9008, -45.0495) (51.4248, -45.2666) (51.8111, -45.6529) knots 0 0 0 0 1 1 1 1
  spline S430 degree 3 poles (54.956, -47.7126) (54.7197, -47.4763) (54.5869, -47.1559) (54.5869, -46.8217) knots 0 0 0 0 1 1 1 1
  spline S431 degree 3 poles (70.73, -34.8747) (71.0515, -34.8747) (71.3487, -34.7031) (71.5094, -34.4247) knots 0 0 0 0 1 1 1 1
  spline S432 degree 3 poles (63.684, -28.9656) (63.4477, -28.7293) (63.315, -28.4088) (63.315, -28.0747) knots 0 0 0 0 1 1 1 1
  line L458 (57.1069, -46.8217) -> (57.1069, -46.8217)
  line L459 (52.4145, -47.1095) -> (52.4145, -47.1095)
  spline S433 degree 3 poles (52.4145, -47.1095) (52.4145, -47.6559) (52.1974, -48.1799) (51.8111, -48.5662) knots 0 0 0 0 1 1 1 1
  spline S434 degree 3 poles (71.5094, -33.5247) (71.3487, -33.2462) (71.0515, -33.0747) (70.73, -33.0747) knots 0 0 0 0 1 1 1 1
  spline S435 degree 3 poles (51.3645, -53.8659) (51.8604, -53.8394) (52.2411, -53.4161) (52.2151, -52.9201) knots 0 0 0 0 1 1 1 1
  spline S436 degree 3 poles (57.1069, -46.8217) (57.1069, -47.1559) (56.9742, -47.4763) (56.7379, -47.7126) knots 0 0 0 0 1 1 1 1
  spline S437 degree 3 poles (129.6216, -61.7615) (129.6216, -61.2973) (129.806, -60.8522) (130.1342, -60.524) knots 0 0 0 0 1 1 1 1
  spline S438 degree 3 poles (71.5094, -34.4247) (71.6702, -34.1462) (71.6702, -33.8031) (71.5094, -33.5247) knots 0 0 0 0 1 1 1 1
  spline S439 degree 3 poles (133.1216, -61.7615) (133.1216, -62.2256) (132.9373, -62.6707) (132.6091, -62.9989) knots 0 0 0 0 1 1 1 1
  spline S440 degree 3 poles (56.7379, -47.7126) (56.5016, -47.9489) (56.1811, -48.0817) (55.8469, -48.0817) knots 0 0 0 0 1 1 1 1
  spline S441 degree 3 poles (132.6091, -62.9989) (132.2809, -63.3271) (131.8358, -63.5115) (131.3716, -63.5115) knots 0 0 0 0 1 1 1 1
  spline S442 degree 3 poles (68.6406, -34.4247) (68.8013, -34.7031) (69.0985, -34.8747) (69.42, -34.8747) knots 0 0 0 0 1 1 1 1
  spline S443 degree 3 poles (65.466, -28.9656) (65.2297, -29.2019) (64.9092, -29.3347) (64.575, -29.3347) knots 0 0 0 0 1 1 1 1
  spline S444 degree 3 poles (65.835, -28.0747) (65.835, -28.4088) (65.7023, -28.7293) (65.466, -28.9656) knots 0 0 0 0 1 1 1 1
  spline S445 degree 3 poles (131.3716, -63.5115) (130.4051, -63.5115) (129.6216, -62.728) (129.6216, -61.7615) knots 0 0 0 0 1 1 1 1
  spline S446 degree 3 poles (43.9711, -48.2883) (43.7348, -48.052) (43.602, -47.7316) (43.602, -47.3974) knots 0 0 0 0 1 1 1 1
  line L460 (70.73, -34.8747) -> (69.42, -34.8747)
  spline S447 degree 3 poles (64.575, -29.3347) (64.2408, -29.3347) (63.9203, -29.2019) (63.684, -28.9656) knots 0 0 0 0 1 1 1 1
  spline S448 degree 3 poles (45.753, -46.5064) (45.9893, -46.7427) (46.122, -47.0632) (46.122, -47.3974) knots 0 0 0 0 1 1 1 1
  line L461 (51.2703, -52.0684) -> (49.962, -52.137)
  spline S449 degree 3 poles (65.466, -27.1837) (65.7023, -27.42) (65.835, -27.7405) (65.835, -28.0747) knots 0 0 0 0 1 1 1 1
  line L462 (65.835, -28.0747) -> (65.835, -28.0747)
  spline S450 degree 3 poles (64.575, -26.8147) (64.9092, -26.8147) (65.2297, -26.9474) (65.466, -27.1837) knots 0 0 0 0 1 1 1 1
  spline S451 degree 3 poles (72.135, -28.0747) (72.135, -28.621) (71.918, -29.145) (71.5316, -29.5313) knots 0 0 0 0 1 1 1 1
  spline S452 degree 3 poles (50.3545, -49.1695) (49.8081, -49.1695) (49.2842, -48.9525) (48.8978, -48.5662) knots 0 0 0 0 1 1 1 1
  spline S453 degree 3 poles (44.862, -48.6574) (44.5278, -48.6574) (44.2073, -48.5246) (43.9711, -48.2883) knots 0 0 0 0 1 1 1 1
  spline S454 degree 3 poles (68.6406, -33.5247) (68.4798, -33.8031) (68.4798, -34.1462) (68.6406, -34.4247) knots 0 0 0 0 1 1 1 1
  line L463 (70.73, -33.0747) -> (69.42, -33.0747)
  spline S455 degree 3 poles (63.315, -28.0747) (63.315, -27.7405) (63.4477, -27.42) (63.684, -27.1837) knots 0 0 0 0 1 1 1 1
  spline S456 degree 3 poles (43.602, -47.3974) (43.602, -47.0632) (43.7348, -46.7427) (43.9711, -46.5064) knots 0 0 0 0 1 1 1 1
  spline S457 degree 3 poles (130.1342, -60.524) (130.4624, -60.1958) (130.9075, -60.0115) (131.3716, -60.0115) knots 0 0 0 0 1 1 1 1
  spline S458 degree 3 poles (45.753, -48.2883) (45.5167, -48.5246) (45.1962, -48.6574) (44.862, -48.6574) knots 0 0 0 0 1 1 1 1
  spline S459 degree 3 poles (54.956, -45.9307) (55.1923, -45.6944) (55.5128, -45.5617) (55.8469, -45.5617) knots 0 0 0 0 1 1 1 1
  spline S460 degree 3 poles (63.684, -27.1837) (63.9203, -26.9474) (64.2408, -26.8147) (64.575, -26.8147) knots 0 0 0 0 1 1 1 1
  spline S461 degree 3 poles (54.5869, -46.8217) (54.5869, -46.4875) (54.7197, -46.167) (54.956, -45.9307) knots 0 0 0 0 1 1 1 1
  spline S462 degree 3 poles (51.8111, -48.5662) (51.4248, -48.9525) (50.9008, -49.1695) (50.3545, -49.1695) knots 0 0 0 0 1 1 1 1
  spline S463 degree 3 poles (48.8978, -45.6529) (49.2842, -45.2666) (49.8081, -45.0495) (50.3545, -45.0495) knots 0 0 0 0 1 1 1 1
  spline S464 degree 3 poles (100.5907, -35.3155) (100.827, -35.0792) (101.1475, -34.9464) (101.4816, -34.9464) knots 0 0 0 0 1 1 1 1
  spline S465 degree 3 poles (108.4349, -37.855) (108.0486, -38.2414) (107.5246, -38.4584) (106.9783, -38.4584) knots 0 0 0 0 1 1 1 1
  spline S466 degree 3 poles (68.015, -28.0747) (68.015, -26.9369) (68.9373, -26.0147) (70.075, -26.0147) knots 0 0 0 0 1 1 1 1
  spline S467 degree 3 poles (106.1149, -20.8654) (105.7286, -20.4791) (105.5116, -19.9551) (105.5116, -19.4087) knots 0 0 0 0 1 1 1 1
  line L464 (88.8426, -53.0853) -> (87.5328, -53.0625)
  spline S468 degree 3 poles (106.9783, -38.4584) (106.4319, -38.4584) (105.908, -38.2414) (105.5217, -37.855) knots 0 0 0 0 1 1 1 1
  spline S469 degree 3 poles (102.9659, -18.3258) (103.2022, -18.5621) (103.3349, -18.8826) (103.3349, -19.2168) knots 0 0 0 0 1 1 1 1
  spline S470 degree 3 poles (103.3349, -19.2168) (103.3349, -19.551) (103.2022, -19.8715) (102.9659, -20.1078) knots 0 0 0 0 1 1 1 1
  line L465 (109.6316, -19.4087) -> (109.6316, -19.4087)
  spline S471 degree 3 poles (105.5217, -34.9418) (105.908, -34.5554) (106.4319, -34.3384) (106.9783, -34.3384) knots 0 0 0 0 1 1 1 1
  line L466 (103.3349, -19.2168) -> (103.3349, -19.2168)
  spline S472 degree 3 poles (94.6651, -49.0616) (94.4288, -49.2979) (94.1083, -49.4306) (93.7742, -49.4306) knots 0 0 0 0 1 1 1 1
  line L467 (114.3282, -19.6007) -> (114.3282, -19.6007)
  spline S473 degree 3 poles (100.8149, -19.2168) (100.8149, -18.8826) (100.9477, -18.5621) (101.184, -18.3258) knots 0 0 0 0 1 1 1 1
  spline S474 degree 3 poles (101.4816, -37.4664) (101.1475, -37.4664) (100.827, -37.3337) (100.5907, -37.0974) knots 0 0 0 0 1 1 1 1
  spline S475 degree 3 poles (109.0383, -36.3984) (109.0383, -36.9447) (108.8213, -37.4687) (108.4349, -37.855) knots 0 0 0 0 1 1 1 1
  spline S476 degree 3 poles (109.0282, -17.9521) (109.4145, -18.3384) (109.6316, -18.8624) (109.6316, -19.4087) knots 0 0 0 0 1 1 1 1
  spline S477 degree 3 poles (108.9191, -25.3594) (108.9364, -24.8629) (108.5482, -24.4463) (108.0517, -24.4286) knots 0 0 0 0 1 1 1 1
  spline S478 degree 3 poles (105.5116, -19.4087) (105.5116, -18.8624) (105.7286, -18.3384) (106.1149, -17.9521) knots 0 0 0 0 1 1 1 1
  spline S479 degree 3 poles (102.0749, -17.9568) (102.4091, -17.9568) (102.7296, -18.0896) (102.9659, -18.3258) knots 0 0 0 0 1 1 1 1
  spline S480 degree 3 poles (92.5142, -48.1706) (92.5142, -47.8365) (92.6469, -47.516) (92.8832, -47.2797) knots 0 0 0 0 1 1 1 1
  spline S481 degree 3 poles (88.8112, -54.885) (89.3079, -54.8932) (89.7172, -54.4975) (89.7259, -54.0009) knots 0 0 0 0 1 1 1 1
  spline S482 degree 3 poles (105.8123, -25.2509) (105.7949, -25.7474) (106.1832, -26.1641) (106.6797, -26.1817) knots 0 0 0 0 1 1 1 1
  spline S483 degree 3 poles (106.7425, -24.3828) (106.246, -24.3659) (105.8296, -24.7544) (105.8123, -25.2509) knots 0 0 0 0 1 1 1 1
  spline S484 degree 3 poles (100.5907, -37.0974) (100.3544, -36.8611) (100.2216, -36.5406) (100.2216, -36.2064) knots 0 0 0 0 1 1 1 1
  spline S485 degree 3 poles (107.9889, -26.2275) (108.4854, -26.2445) (108.9017, -25.8559) (108.9191, -25.3594) knots 0 0 0 0 1 1 1 1
  spline S486 degree 3 poles (102.3726, -37.0974) (102.1363, -37.3337) (101.8158, -37.4664) (101.4816, -37.4664) knots 0 0 0 0 1 1 1 1
  spline S487 degree 3 poles (109.6316, -19.4087) (109.6316, -19.9551) (109.4145, -20.4791) (109.0282, -20.8654) knots 0 0 0 0 1 1 1 1
  spline S488 degree 3 poles (105.5217, -37.855) (105.1353, -37.4687) (104.9183, -36.9447) (104.9183, -36.3984) knots 0 0 0 0 1 1 1 1
  spline S489 degree 3 poles (112.1773, -18.7097) (112.4136, -18.4734) (112.7341, -18.3407) (113.0682, -18.3407) knots 0 0 0 0 1 1 1 1
  spline S490 degree 3 poles (111.8082, -19.6007) (111.8082, -19.2665) (111.941, -18.946) (112.1773, -18.7097) knots 0 0 0 0 1 1 1 1
  spline S491 degree 3 poles (102.9659, -20.1078) (102.7296, -20.3441) (102.4091, -20.4768) (102.0749, -20.4768) knots 0 0 0 0 1 1 1 1
  spline S492 degree 3 poles (101.184, -20.1078) (100.9477, -19.8715) (100.8149, -19.551) (100.8149, -19.2168) knots 0 0 0 0 1 1 1 1
  spline S493 degree 3 poles (95.0342, -48.1706) (95.0342, -48.5048) (94.9014, -48.8253) (94.6651, -49.0616) knots 0 0 0 0 1 1 1 1
  spline S494 degree 3 poles (104.9183, -36.3984) (104.9183, -35.852) (105.1353, -35.3281) (105.5217, -34.9418) knots 0 0 0 0 1 1 1 1
  line L468 (107.9889, -26.2275) -> (106.6797, -26.1817)
  spline S495 degree 3 poles (107.5716, -21.4687) (107.0252, -21.4687) (106.5013, -21.2517) (106.1149, -20.8654) knots 0 0 0 0 1 1 1 1
  spline S496 degree 3 poles (112.1773, -20.4916) (111.941, -20.2554) (111.8082, -19.9349) (111.8082, -19.6007) knots 0 0 0 0 1 1 1 1
  spline S497 degree 3 poles (113.0682, -20.8607) (112.7341, -20.8607) (112.4136, -20.7279) (112.1773, -20.4916) knots 0 0 0 0 1 1 1 1
  spline S498 degree 3 poles (107.5716, -17.3487) (108.1179, -17.3487) (108.6419, -17.5658) (109.0282, -17.9521) knots 0 0 0 0 1 1 1 1
  spline S499 degree 3 poles (113.9592, -18.7097) (114.1955, -18.946) (114.3282, -19.2665) (114.3282, -19.6007) knots 0 0 0 0 1 1 1 1
  spline S500 degree 3 poles (101.184, -18.3258) (101.4203, -18.0896) (101.7408, -17.9568) (102.0749, -17.9568) knots 0 0 0 0 1 1 1 1
  spline S501 degree 3 poles (86.6181, -53.9466) (86.6095, -54.4433) (87.0048, -54.853) (87.5014, -54.8622) knots 0 0 0 0 1 1 1 1
  spline S502 degree 3 poles (87.5328, -53.0625) (87.0362, -53.0543) (86.6268, -53.45) (86.6181, -53.9466) knots 0 0 0 0 1 1 1 1
  line L469 (88.8112, -54.8851) -> (87.5014, -54.8622)
  spline S503 degree 3 poles (92.8832, -49.0616) (92.6469, -48.8253) (92.5142, -48.5048) (92.5142, -48.1706) knots 0 0 0 0 1 1 1 1
  spline S504 degree 3 poles (102.3726, -35.3155) (102.6089, -35.5518) (102.7416, -35.8723) (102.7416, -36.2064) knots 0 0 0 0 1 1 1 1
  spline S505 degree 3 poles (113.0682, -18.3407) (113.4024, -18.3407) (113.7229, -18.4734) (113.9592, -18.7097) knots 0 0 0 0 1 1 1 1
  spline S506 degree 3 poles (102.0749, -20.4768) (101.7408, -20.4768) (101.4203, -20.3441) (101.184, -20.1078) knots 0 0 0 0 1 1 1 1
  spline S507 degree 3 poles (106.1149, -17.9521) (106.5013, -17.5658) (107.0252, -17.3487) (107.5716, -17.3487) knots 0 0 0 0 1 1 1 1
  spline S508 degree 3 poles (113.9592, -20.4916) (113.7229, -20.7279) (113.4024, -20.8607) (113.0682, -20.8607) knots 0 0 0 0 1 1 1 1
  spline S509 degree 3 poles (106.9783, -34.3384) (108.116, -34.3384) (109.0383, -35.2607) (109.0383, -36.3984) knots 0 0 0 0 1 1 1 1
  spline S510 degree 3 poles (93.7742, -49.4306) (93.44, -49.4306) (93.1195, -49.2979) (92.8832, -49.0616) knots 0 0 0 0 1 1 1 1
  spline S511 degree 3 poles (100.2216, -36.2064) (100.2216, -35.8723) (100.3544, -35.5518) (100.5907, -35.3155) knots 0 0 0 0 1 1 1 1
  line L470 (102.7416, -36.2064) -> (102.7416, -36.2064)
  line L471 (109.0383, -36.3984) -> (109.0383, -36.3984)
  spline S512 degree 3 poles (114.3282, -19.6007) (114.3282, -19.9349) (114.1955, -20.2554) (113.9592, -20.4916) knots 0 0 0 0 1 1 1 1
  spline S513 degree 3 poles (89.7259, -54.0009) (89.7346, -53.5042) (89.3393, -53.0945) (88.8426, -53.0853) knots 0 0 0 0 1 1 1 1
  spline S514 degree 3 poles (109.0282, -20.8654) (108.6419, -21.2517) (108.1179, -21.4687) (107.5716, -21.4687) knots 0 0 0 0 1 1 1 1
  spline S515 degree 3 poles (92.8832, -47.2797) (93.1195, -47.0434) (93.44, -46.9106) (93.7742, -46.9106) knots 0 0 0 0 1 1 1 1
  spline S516 degree 3 poles (93.7742, -46.9106) (94.1083, -46.9106) (94.4288, -47.0434) (94.6651, -47.2797) knots 0 0 0 0 1 1 1 1
  line L472 (108.0517, -24.4286) -> (106.7425, -24.3828)
  spline S517 degree 3 poles (101.4816, -34.9464) (101.8158, -34.9464) (102.1363, -35.0792) (102.3726, -35.3155) knots 0 0 0 0 1 1 1 1
  spline S518 degree 3 poles (68.6184, -29.5313) (68.232, -29.145) (68.015, -28.621) (68.015, -28.0747) knots 0 0 0 0 1 1 1 1
  spline S519 degree 3 poles (83.6668, -47.0877) (83.9031, -47.324) (84.0358, -47.6445) (84.0358, -47.9787) knots 0 0 0 0 1 1 1 1
  spline S520 degree 3 poles (89.7316, -46.618) (90.118, -47.0043) (90.335, -47.5283) (90.335, -48.0747) knots 0 0 0 0 1 1 1 1
  spline S521 degree 3 poles (101.4716, -5.2515) (101.9358, -5.2515) (102.3809, -5.4358) (102.7091, -5.764) knots 0 0 0 0 1 1 1 1
  spline S522 degree 3 poles (50.9214, -31.5895) (50.5351, -31.9758) (50.0111, -32.1928) (49.4648, -32.1928) knots 0 0 0 0 1 1 1 1
  spline S523 degree 3 poles (49.4648, -32.1928) (48.9184, -32.1928) (48.3944, -31.9758) (48.0081, -31.5895) knots 0 0 0 0 1 1 1 1
  spline S524 degree 3 poles (50.4747, -36.8892) (50.9707, -36.8627) (51.3514, -36.4394) (51.3254, -35.9434) knots 0 0 0 0 1 1 1 1
  spline S525 degree 3 poles (82.7758, -49.2387) (82.4417, -49.2387) (82.1212, -49.1059) (81.8849, -48.8696) knots 0 0 0 0 1 1 1 1
  line L473 (90.335, -48.0747) -> (90.335, -48.0747)
  spline S526 degree 3 poles (101.4716, -8.7515) (100.5051, -8.7515) (99.7216, -7.968) (99.7216, -7.0015) knots 0 0 0 0 1 1 1 1
  spline S527 degree 3 poles (54.0663, -30.7359) (53.83, -30.4996) (53.6972, -30.1792) (53.6972, -29.845) knots 0 0 0 0 1 1 1 1
  line L474 (45.2323, -30.4207) -> (45.2323, -30.4207)
  spline S528 degree 3 poles (90.335, -48.0747) (90.335, -48.621) (90.118, -49.145) (89.7316, -49.5313) knots 0 0 0 0 1 1 1 1
  spline S529 degree 3 poles (84.0358, -47.9787) (84.0358, -48.3128) (83.9031, -48.6333) (83.6668, -48.8696) knots 0 0 0 0 1 1 1 1
  spline S530 degree 3 poles (86.8184, -46.618) (87.2047, -46.2317) (87.7287, -46.0147) (88.275, -46.0147) knots 0 0 0 0 1 1 1 1
  spline S531 degree 3 poles (83.6668, -48.8696) (83.4305, -49.1059) (83.11, -49.2387) (82.7758, -49.2387) knots 0 0 0 0 1 1 1 1
  spline S532 degree 3 poles (42.7123, -30.4207) (42.7123, -30.0865) (42.845, -29.766) (43.0813, -29.5297) knots 0 0 0 0 1 1 1 1
  spline S533 degree 3 poles (99.7216, -7.0015) (99.7216, -6.035) (100.5051, -5.2515) (101.4716, -5.2515) knots 0 0 0 0 1 1 1 1
  spline S534 degree 3 poles (94.6651, -47.2797) (94.9014, -47.516) (95.0342, -47.8365) (95.0342, -48.1706) knots 0 0 0 0 1 1 1 1
  spline S535 degree 3 poles (49.0723, -35.1603) (48.5764, -35.1868) (48.1957, -35.6101) (48.2217, -36.1061) knots 0 0 0 0 1 1 1 1
  spline S536 degree 3 poles (43.9723, -31.6807) (43.6381, -31.6807) (43.3176, -31.5479) (43.0813, -31.3116) knots 0 0 0 0 1 1 1 1
  spline S537 degree 3 poles (44.8633, -29.5297) (45.0996, -29.766) (45.2323, -30.0865) (45.2323, -30.4207) knots 0 0 0 0 1 1 1 1
  spline S538 degree 3 poles (54.9572, -28.585) (55.2914, -28.585) (55.6119, -28.7177) (55.8482, -28.954) knots 0 0 0 0 1 1 1 1
  spline S539 degree 3 poles (82.7758, -46.7187) (83.11, -46.7187) (83.4305, -46.8514) (83.6668, -47.0877) knots 0 0 0 0 1 1 1 1
  spline S540 degree 3 poles (43.9723, -29.1607) (44.3065, -29.1607) (44.627, -29.2934) (44.8633, -29.5297) knots 0 0 0 0 1 1 1 1
  line L475 (103.2216, -7.0015) -> (103.2216, -7.0015)
  line L476 (95.0342, -48.1706) -> (95.0342, -48.1706)
  spline S541 degree 3 poles (44.8633, -31.3116) (44.627, -31.5479) (44.3065, -31.6807) (43.9723, -31.6807) knots 0 0 0 0 1 1 1 1
  spline S542 degree 3 poles (55.8482, -30.7359) (55.6119, -30.9722) (55.2914, -31.105) (54.9572, -31.105) knots 0 0 0 0 1 1 1 1
  spline S543 degree 3 poles (53.6972, -29.845) (53.6972, -29.5108) (53.83, -29.1903) (54.0663, -28.954) knots 0 0 0 0 1 1 1 1
  line L477 (50.4747, -36.8892) -> (49.1665, -36.9578)
  spline S544 degree 3 poles (103.2216, -7.0015) (103.2216, -7.4656) (103.0373, -7.9107) (102.7091, -8.2389) knots 0 0 0 0 1 1 1 1
  spline S545 degree 3 poles (45.2323, -30.4207) (45.2323, -30.7549) (45.0996, -31.0753) (44.8633, -31.3116) knots 0 0 0 0 1 1 1 1
  spline S546 degree 3 poles (54.0663, -28.954) (54.3026, -28.7177) (54.6231, -28.585) (54.9572, -28.585) knots 0 0 0 0 1 1 1 1
  spline S547 degree 3 poles (88.275, -46.0147) (88.8213, -46.0147) (89.3453, -46.2317) (89.7316, -46.618) knots 0 0 0 0 1 1 1 1
  line L478 (56.2172, -29.845) -> (56.2172, -29.845)
  line L479 (84.0358, -47.9787) -> (84.0358, -47.9787)
  spline S548 degree 3 poles (48.0081, -31.5895) (47.6218, -31.2032) (47.4048, -30.6792) (47.4048, -30.1328) knots 0 0 0 0 1 1 1 1
  spline S549 degree 3 poles (102.7416, -36.2064) (102.7416, -36.5406) (102.6089, -36.8611) (102.3726, -37.0974) knots 0 0 0 0 1 1 1 1
  spline S550 degree 3 poles (56.2172, -29.845) (56.2172, -30.1792) (56.0845, -30.4996) (55.8482, -30.7359) knots 0 0 0 0 1 1 1 1
  spline S551 degree 3 poles (47.4048, -30.1328) (47.4048, -28.9951) (48.3271, -28.0728) (49.4648, -28.0728) knots 0 0 0 0 1 1 1 1
  spline S552 degree 3 poles (49.4648, -28.0728) (50.0111, -28.0728) (50.5351, -28.2899) (50.9214, -28.6762) knots 0 0 0 0 1 1 1 1
  spline S553 degree 3 poles (86.215, -48.0747) (86.215, -47.5283) (86.432, -47.0043) (86.8184, -46.618) knots 0 0 0 0 1 1 1 1
  line L480 (51.5248, -30.1328) -> (51.5248, -30.1328)
  spline S554 degree 3 poles (50.9214, -28.6762) (51.3077, -29.0625) (51.5248, -29.5865) (51.5248, -30.1328) knots 0 0 0 0 1 1 1 1
  spline S555 degree 3 poles (81.5158, -47.9787) (81.5158, -47.6445) (81.6486, -47.324) (81.8849, -47.0877) knots 0 0 0 0 1 1 1 1
  spline S556 degree 3 poles (86.8184, -49.5313) (86.432, -49.145) (86.215, -48.621) (86.215, -48.0747) knots 0 0 0 0 1 1 1 1
  line L481 (50.3805, -35.0917) -> (49.0723, -35.1603)
  spline S557 degree 3 poles (89.7316, -49.5313) (89.3453, -49.9176) (88.8213, -50.1347) (88.275, -50.1347) knots 0 0 0 0 1 1 1 1
  spline S558 degree 3 poles (81.8849, -48.8696) (81.6486, -48.6333) (81.5158, -48.3128) (81.5158, -47.9787) knots 0 0 0 0 1 1 1 1
  spline S559 degree 3 poles (113.3659, -35.6994) (113.6022, -35.9357) (113.7349, -36.2562) (113.7349, -36.5903) knots 0 0 0 0 1 1 1 1
  spline S560 degree 3 poles (48.2217, -36.1061) (48.2477, -36.6021) (48.6705, -36.9832) (49.1665, -36.9578) knots 0 0 0 0 1 1 1 1